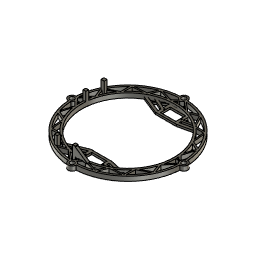
Lower_Bulkhead (Autodesk Fusion 360 design; units mm, degrees)
Autodesk Fusion 360 part; units mm, degrees
note: some values were not read from the file. Set by a fixed rule: which sketch regions a step uses.
sketch "Sketch1" plane through (0, 0, 0) normal (0, 0, 1) x (1, 0, 0)
  circle A0 centre (-87, 0) radius 3.5
  circle A1 centre (-87, 0) radius 6
  circle A2 centre (0, -87) radius 6
  circle A3 centre (0, -87) radius 3.5
  circle A4 centre (87, 0) radius 6
  circle A5 centre (87, 0) radius 3.5
  circle A6 centre (0, 87) radius 6
  circle A7 centre (0, 87) radius 3.5
  circle A8 centre (0, 0) radius 87
  circle A9 centre (0, 0) radius 75
  circle A10 centre (0, 0) radius 72
  circle A11 centre (0, 0) radius 84
  line L0 (-81.0415, -0.7044) -> (-74.9967, -0.7044)
  line L1 (-81.053, 0.7956) -> (-74.9958, 0.7956)
  line L2 (0.7044, -81.0415) -> (0.7044, -74.9967)
  line L3 (-0.7956, -81.053) -> (-0.7956, -74.9958)
  line L4 (81.0415, 0.7044) -> (74.9967, 0.7044)
  line L5 (81.053, -0.7956) -> (74.9958, -0.7956)
  line L6 (-0.7044, 81.0415) -> (-0.7044, 74.9967)
  line L7 (0.7956, 81.053) -> (0.7956, 74.9958)
  line L8 (-83.708, 6.9977) -> (-72.0178, 20.9389)
  line L9 (-83.1247, 4.5806) -> (-73.1745, 16.4468)
  line L10 (-78.5501, -27.5785) -> (-73.8983, -12.8078)
  line L11 (-80.014, -25.5687) -> (-74.5487, -8.215)
  line L12 (-62.017, -55.5391) -> (-63.3718, -40.1125)
  line L13 (-64.1386, -54.2424) -> (-65.7303, -36.1182)
  line L14 (-36.0424, -75.0443) -> (-43.1975, -61.3105)
  line L15 (-38.4987, -74.6582) -> (-46.905, -58.5228)
  line L16 (-4.5806, -83.1247) -> (-16.4468, -73.1745)
  line L17 (-6.9977, -83.708) -> (-20.9389, -72.0178)
  line L18 (27.5785, -78.5501) -> (12.8078, -73.8983)
  line L19 (25.5687, -80.014) -> (8.215, -74.5487)
  line L20 (55.5391, -62.017) -> (40.1125, -63.3718)
  line L21 (54.2424, -64.1386) -> (36.1182, -65.7303)
  line L22 (75.0443, -36.0424) -> (61.3105, -43.1975)
  line L23 (74.6582, -38.4987) -> (58.5228, -46.905)
  line L24 (83.1247, -4.5806) -> (73.1745, -16.4468)
  line L25 (83.708, -6.9977) -> (72.0178, -20.9389)
  line L26 (78.5501, 27.5785) -> (73.8983, 12.8078)
  line L27 (80.014, 25.5687) -> (74.5487, 8.215)
  line L28 (62.017, 55.5391) -> (63.3718, 40.1125)
  line L29 (64.1386, 54.2424) -> (65.7303, 36.1182)
  line L30 (36.0424, 75.0443) -> (43.1975, 61.3105)
  line L31 (38.4987, 74.6582) -> (46.905, 58.5228)
  line L32 (4.5806, 83.1247) -> (16.4468, 73.1745)
  line L33 (6.9977, 83.708) -> (20.9389, 72.0178)
  line L34 (-27.5785, 78.5501) -> (-12.8078, 73.8983)
  line L35 (-25.5687, 80.014) -> (-8.215, 74.5487)
  line L36 (-55.5391, 62.017) -> (-40.1125, 63.3718)
  line L37 (-54.2424, 64.1386) -> (-36.1182, 65.7303)
  line L38 (-75.0443, 36.0424) -> (-61.3105, 43.1975)
  line L39 (-74.6582, 38.4987) -> (-58.5228, 46.905)
  line L40 (-72.0178, 20.9389) -> (-77.0162, 33.5337)
  line L41 (-70.8151, 24.7028) -> (-75.0443, 36.0424)
  line L42 (-74.8779, -4.2774) -> (-83.1247, 4.5806)
  line L43 (-74.5487, -8.215) -> (-83.9865, 1.5083)
  line L44 (-67.5413, -32.6063) -> (-78.5501, -27.5785)
  line L45 (-65.7303, -36.1182) -> (-78.1706, -30.7467)
  line L46 (-49.9221, -55.9712) -> (-62.017, -55.5391)
  line L47 (-46.905, -58.5228) -> (-60.4539, -58.3209)
  line L48 (-24.7028, -70.8151) -> (-36.0424, -75.0443)
  line L49 (-20.9389, -72.0178) -> (-33.5337, -77.0162)
  line L50 (4.2774, -74.8779) -> (-4.5806, -83.1247)
  line L51 (8.215, -74.5487) -> (-1.5083, -83.9865)
  line L52 (32.6063, -67.5413) -> (27.5785, -78.5501)
  line L53 (36.1182, -65.7303) -> (30.7467, -78.1706)
  line L54 (55.9712, -49.9221) -> (55.5391, -62.017)
  line L55 (58.5228, -46.905) -> (58.3209, -60.4539)
  line L56 (70.8151, -24.7028) -> (75.0443, -36.0424)
  line L57 (72.0178, -20.9389) -> (77.0162, -33.5337)
  line L58 (74.8779, 4.2774) -> (83.1247, -4.5806)
  line L59 (74.5487, 8.215) -> (83.9865, -1.5083)
  line L60 (67.5413, 32.6063) -> (78.5501, 27.5785)
  line L61 (65.7303, 36.1182) -> (78.1706, 30.7467)
  line L62 (49.9221, 55.9712) -> (62.017, 55.5391)
  line L63 (46.905, 58.5228) -> (60.4539, 58.3209)
  line L64 (24.7028, 70.8151) -> (36.0424, 75.0443)
  line L65 (20.9389, 72.0178) -> (33.5337, 77.0162)
  line L66 (-4.2774, 74.8779) -> (4.5806, 83.1247)
  line L67 (-8.215, 74.5487) -> (1.5083, 83.9865)
  line L68 (-32.6063, 67.5413) -> (-27.5785, 78.5501)
  line L69 (-36.1182, 65.7303) -> (-30.7467, 78.1706)
  line L70 (-55.9712, 49.9221) -> (-55.5391, 62.017)
  line L71 (-58.5228, 46.905) -> (-58.3209, 60.4539)
  line L72 (-71.0817, 10.2586) -> (-76.0817, 10.2586)
  line L73 (-76.0817, 5.9336) -> (-76.0817, 10.2586)
  line L74 (-71.0817, 10.2586) -> (-71.0817, 5.9336)
  line L75 (-71.0817, 5.9336) -> (-76.0817, 5.9336)
  line L76 (-71.0817, 38.4656) -> (-76.0817, 38.4656)
  line L77 (-76.0817, 38.4656) -> (-76.0817, 34.1406)
  line L78 (-76.0817, 34.1406) -> (-71.0817, 34.1406)
  line L79 (-71.0817, 34.1406) -> (-71.0817, 38.4656)
  line L80 (-34.1406, -71.0817) -> (-38.4656, -71.0817)
  line L81 (-38.4656, -71.0817) -> (-38.4656, -76.0817)
  line L82 (-38.4656, -76.0817) -> (-34.1406, -76.0817)
  line L83 (-34.1406, -76.0817) -> (-34.1406, -71.0817)
  line L84 (-10.2586, -71.0817) -> (-10.2586, -76.0817)
  line L85 (-10.2586, -71.0817) -> (-5.9336, -71.0817)
  line L86 (-5.9336, -71.0817) -> (-5.9336, -76.0817)
  line L87 (-5.9336, -76.0817) -> (-10.2586, -76.0817)
  dimension "d1" = 87
  dimension "d2" = 12
  dimension "d3" = 7
  dimension "d5" = 360
  dimension "d6" = 150
  dimension "d7" = 3
  dimension "d8" = 3
  dimension "d9" = 1.5
  dimension "d11" = 360
  dimension "d12" = 2
  dimension "d14" = 360
  dimension "d15" = 1.193
  dimension "d17" = 360
  constraint concentric A0 A1
  constraint coincident A8.centre A9.centre
  constraint coincident A4.centre A8
  constraint concentric A9 A10
  constraint concentric A8 A11
  constraint coincident A1 L0.start
  constraint coincident A9 L0.end
  constraint horizontal L0
  constraint coincident A1 L1.start
  constraint coincident A9 L1.end
  constraint parallel L0 L1
  constraint coincident A11 L8.start
  constraint coincident A9 L8.end
  constraint coincident A1 L9.start
  constraint coincident A9 L9.end
  constraint parallel L8 L9
  constraint coincident A11 L40.end
  constraint coincident A9 L41.start
  constraint perpendicular L74 L75
  measures "d1" distance of A8.centre A0.centre
  measures "d2" diameter of A1
  measures "d3" diameter of A0
  measures "d6" diameter of A9
  measures "d7" distance of A9 A10
  measures "d8" distance of A8 A11
  measures "d9" distance of L0 L1
  measures "d12" distance of L8 L9
  measures "d15" angle of L40 L41
extrude "Extrude1" add sketch "Sketch1" along normal blind 7 contours A0 A1 A11 L43 | A0 A1 A11 L42 L43 | A0 A1 A8 A11 | A0 A1 A8 A11 | A1 A9 L0 L42 L43 | A0 A1 A8 | A1 A2 A8 A11 L81 L82 | A1 A9 A11 L8 L9 | A1 A6 A8 A11 L76 L77 | A1 L0 L1 L42 | A9 A10 L75 L84 | A9 A11 L10 L11 L44 L45 | A9 L0 L1 L42 | A2 A3 A8 | A2 A3 A8 A11 | A6 A7 A8 A11 | A6 A7 A8 | A1 L1 L42 | A9 A10 L72 L86 | A9 A11 L40 L41 L77 L78 | A2 A9 A11 L16 L17 | A2 A3 A11 L50 L51 | A9 A11 L12 L13 L46 L47 | A6 A7 A11 L67 | A9 A10 L72 L75 | A11 L76 L77 | A11 L38 L41 L76 L77 L78 L79 | A2 A3 A8 A11 | A2 A4 A8 A11 | A4 A6 A8 A11 | A6 A7 A8 A11 | A6 A7 A11 L66 L67 | A6 A9 L6 L66 L67 | A9 A11 L34 L35 L68 L69 | A9 A11 L38 L39 L76 L79 | A2 L3 L50 | A9 A11 L48 L49 L82 L83 | A2 A3 A11 L51 | A4 A5 A8 | A4 A5 A8 A11 | A9 A11 L14 L15 L80 L81 | A6 A9 A11 L32 L33 | A4 A5 A8 A11 | A6 L6 L7 L66 | A9 A11 L36 L37 L70 L71 | A2 L2 L3 L50 | A9 L2 L3 L50 | A9 A10 L84 L86 | A11 L81 L82 | A11 L14 L48 L80 L81 L82 L83 | A2 A9 L2 L50 L51 | A9 A11 L18 L19 L52 L53 | A4 A9 A11 L24 L25 | A4 A5 A11 L58 L59 | A4 A5 A11 L59 | A6 L7 L66 | A9 L6 L7 L66 | A9 A11 L30 L31 L64 L65 | A4 A9 L4 L58 L59 | A9 A11 L26 L27 L60 L61 | A9 A11 L20 L21 L54 L55 | A9 A11 L22 L23 L56 L57 | A9 L4 L5 L58 | A9 A11 L28 L29 L62 L63 makes body 1
extrude "Extrude2" add sketch "Sketch1" along normal blind 21 contours A9 A10 L72 L75 | A9 L72 L73 L75 | A11 L76 L77 | A11 L38 L41 L76 L77 L78 L79 | L38 L41 L78 L79 | A9 A10 L84 L86 | A9 L84 L86 L87 | A11 L81 L82 | A11 L14 L48 L80 L81 L82 L83 | L14 L48 L80 L83 bodies 1
sketch "Sketch2" plane through (0, 0, 0) normal (0, 0, 1) x (1, 0, 0)
  line L0 (20.8629, -68.5916) -> (-3.0191, -68.5916)
  line L1 (-3.0191, -68.5916) -> (-3.0191, -63.5916)
  line L2 (-3.0191, -63.5916) -> (-3.0191, -53.5916)
  line L3 (-3.0191, -53.5916) -> (20.8629, -53.5916)
  line L4 (20.8629, -63.5916) -> (20.8629, -53.5916)
  line L5 (20.8629, -63.5916) -> (20.8629, -68.5916)
  circle A0 centre (22.6129, -61.0916) radius 1.038
  circle A1 centre (-4.7591, -61.0916) radius 1.038
  line L6 (1.75, 0) -> (22.5, 0)
  line L7 (20.8629, 63.5916) -> (20.8629, 68.5916)
  line L8 (-3.0191, 68.5916) -> (-3.0191, 63.5916)
  line L9 (-3.0191, 63.5916) -> (-3.0191, 53.5916)
  line L10 (-3.0191, 53.5916) -> (20.8629, 53.5916)
  line L11 (20.8629, 68.5916) -> (-3.0191, 68.5916)
  circle A2 centre (-4.7591, 61.0916) radius 1.038
  line L12 (20.8629, 63.5916) -> (20.8629, 53.5916)
  circle A3 centre (22.6129, 61.0916) radius 1.038
  line L13 (-3.0191, 68.5916) -> (-3.0191, 72.8205)
  line L14 (-3.0191, 72.8205) -> (-7.6855, 72.8205)
  line L15 (-7.6855, 72.8205) -> (-7.6855, 50.1356)
  line L16 (-7.6855, 50.1356) -> (25.1142, 50.1356)
  line L17 (25.1142, 50.1356) -> (25.1142, 68.5916)
  line L18 (-7.6855, 50.1356) -> (-40.1519, 63.2207)
  line L19 (-40.1519, 63.2207) -> (-36.1256, 65.6758)
  line L20 (-36.1256, 65.6758) -> (-7.6855, 54.2134)
  line L21 (-26.5023, 61.7972) -> (-7.6855, 74.514)
  line L22 (-7.6855, 74.514) -> (-4.4061, 74.514)
  line L23 (-4.4061, 74.514) -> (-24.448, 60.9693)
  line L24 (-7.6855, 58.8998) -> (-26.8946, 67.7416)
  line L25 (-26.8946, 67.7416) -> (-23.3797, 70.1171)
  line L26 (-23.3797, 70.1171) -> (-7.6855, 62.8931)
  line L27 (25.1142, 50.1356) -> (49.6969, 55.6707)
  line L28 (49.6969, 55.6707) -> (46.4863, 59.3636)
  line L29 (46.4863, 59.3636) -> (25.1142, 54.5514)
  line L30 (25.1142, 57.9182) -> (39.9132, 61.2504)
  line L31 (39.9132, 61.2504) -> (37.682, 63.8167)
  line L32 (37.682, 63.8167) -> (25.1142, 60.9869)
  line L33 (-7.6855, 72.8205) -> (19.2542, 72.8205)
  line L34 (19.2542, 72.8205) -> (25.1142, 68.5916)
  dimension "d58" = 15
  dimension "d59" = 23.882
  dimension "d73" = 2.076
  dimension "d74" = 2.076
  dimension "d75" = 7.5
  dimension "d76" = 7.5
  dimension "d77" = 1.74
  dimension "d78" = 1.75
  constraint perpendicular L2 L3
  constraint perpendicular L3 L4
  constraint symmetric L0.start L6 L7.end
  constraint symmetric L3.end L6 L10.end
  constraint symmetric L1.end L6 L8.end
  constraint symmetric L2.end L6 L9.end
  constraint symmetric L0.end L6 L8.start
  constraint symmetric L4.start L6 L7.start
  constraint symmetric A0 L6 A3
  constraint symmetric A1 L6 A2
  constraint perpendicular L11 L13
  constraint perpendicular L13 L14
  constraint perpendicular L11 L15
  constraint perpendicular L13 L16
  constraint perpendicular L11 L17
  constraint coincident L15 L20.end
  constraint parallel L18 L20
  constraint coincident L20 L21.start
  constraint perpendicular L15 L22
  constraint coincident L20 L23.end
  constraint parallel L21 L23
  constraint coincident L15 L24.start
  constraint parallel L21 L25
  constraint coincident L15 L26.end
  constraint parallel L24 L26
  constraint coincident L17 L29.end
  constraint parallel L27 L29
  constraint coincident L17 L30.start
  constraint parallel L29 L30
  constraint parallel L28 L31
  constraint coincident L17 L32.end
  constraint parallel L30 L32
  constraint perpendicular L15 L33
  measures "d58" distance of L0 L3
  measures "d59" distance of L2 L4
  measures "d73" diameter of A1
  measures "d74" diameter of A0
  measures "d75" distance of A0.centre L3
  measures "d76" distance of A1.centre L3
  measures "d77" distance of A1.centre L2
  measures "d78" distance of A0.centre L4
extrude "Extrude3" add sketch "Sketch2" along normal blind 3 separate body contours L14 L15 L16 L17 L23 L33 L34 | L14 L15 L21 L22 L23 L26 L33 | L15 L23 L24 L26 | L21 L23 L24 L26 | L17 L30 L31 L32 | L21 L24 L25 L26 | L20 L21 L23 L24 | L15 L18 L19 L20 | L17 L27 L28 L29 makes body 2
mirror "Mirror1" about plane through (0, 0, 0) normal (0, 1, 0) of bodies 2 makes body 3
ref_plane "WorkPlane2" through (-8.0961, -76.0817, 10.5) normal (0, -1, 0) x (1, 0, 0)
sketch "Sketch4" plane through (-8.0961, -76.0817, 10) normal (0, -1, 0) x (1, 0, 0)
  line L0 (2.1176, 9.9366) -> (22.1566, -3.9365)
  line L1 (22.1566, -3.9365) -> (2.1176, -3.9365)
  line L2 (2.1176, -3.9365) -> (2.1176, 9.9366)
  constraint horizontal L1
  constraint perpendicular L1 L2
extrude "Extrude4" add sketch "Sketch4" against normal blind 4 bodies 1
sketch "Sketch5" plane through (-60.8722, -31.7137, 0) normal (-0.886858, -0.462042, 0) x (0.462042, -0.886858, 0)
  line L0 (30.2293, 0) -> (48.4233, 0)
  line L1 (48.4233, 0) -> (48.4233, 7)
  line L2 (48.4233, 7) -> (30.2293, 7)
  line L3 (30.2293, 7) -> (30.2293, 0)
  line L4 (49.6578, 20.9399) -> (30.2293, 7)
  line L5 (30.2293, 7) -> (49.6578, 7)
  line L6 (49.6578, 7) -> (49.6578, 20.9399)
  constraint coincident L2.end L3.start
  constraint perpendicular L3 L5
  constraint perpendicular L5 L6
extrude "Extrude5" add sketch "Sketch5" against normal blind 2 contours L2 L4 L5 L6 bodies 1
